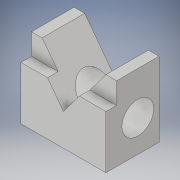
# Autodesk Inventor part: P3-11
Saved by Autodesk Inventor 2017 (Build 210142000, 142)
## iProperties
Created: 2017-02-12
Part Number: P3-11
Material: Generic
Document SubType Name: Modeling
Designer: Schaffel
Density: 1 g/cm^3
Appearance: Default
Author: Schaffel
Autodesk Inventor part; units mm, degrees
ref_plane "YZ Plane" through (0, 0, 0) normal (1, 0, 0) x (0, 1, 0)
ref_plane "XZ Plane" through (0, 0, 0) normal (0, 1, 0) x (-1, 0, 0)
ref_plane "XY Plane" through (0, 0, 0) normal (0, 0, 1) x (1, 0, 0)
sketch "Sketch1" plane through (0, 0, 0) normal (0, 0, 1) x (1, 0, 0)
  line L0 (0, 0) -> (101.6, 0)
  line L1 (101.6, 0) -> (101.6, 88.9)
  line L2 (101.6, 88.9) -> (0, 88.9)
  line L3 (0, 88.9) -> (0, 0)
  dimension "d0" = 101.6
  dimension "d1" = 88.9
  constraints: 8 end point, 3 perpendicular, 1 horizontal
  measures "d0" distance of L0.start L0.end
  measures "d1" distance of L0.end L1.end
extrude "Extrusion1" add sketch "Sketch1" along normal blind 63.5
sketch "Sketch2" plane through (0, 0, 63.5) normal (0, 0, 1) x (1, 0, 0)
  line L0 (101.6, 88.9) -> (88.9, 88.9)
  line L1 (88.9, 88.9) -> (50.8, 38.1)
  line L2 (12.7, 88.9) -> (50.8, 38.1)
  line L3 (12.7, 88.9) -> (88.9, 88.9)
  line L4 (101.6, 88.9) -> (0, 88.9) projected
  point P0 (0, 0)
  constraints: 8 end point, 1 collinear, 1 point on line
extrude "Extrusion2" cut sketch "Sketch2" against normal blind 63.5
sketch "Sketch3" plane through (101.6, 0, 0) normal (1, 0, 0) x (0, 0, -1)
  line L0 (0, 88.9) -> (-63.5, 88.9) projected
  line L1 (-63.5, 88.9) -> (-50.8, 88.9)
  line L2 (-50.8, 63.5) -> (-63.5, 63.5)
  line L3 (-63.5, 0) -> (-63.5, 88.9) projected
  line L4 (-63.5, 63.5) -> (-63.5, 88.9)
  line L5 (-50.8, 88.9) -> (-50.8, 63.5)
  line L6 (-63.5, 38.1) -> (0, 38.1) projected
  circle A0 centre (-25.4, 38.1) radius 19.05
  point P0 (0, 0)
  constraints: 8 end point, 2 point on line, 1 centre point, 1 collinear, 1 horizontal, 1 perpendicular
extrude "Extrusion3" cut sketch "Sketch3" against normal blind 101.6
body "Solid1"
